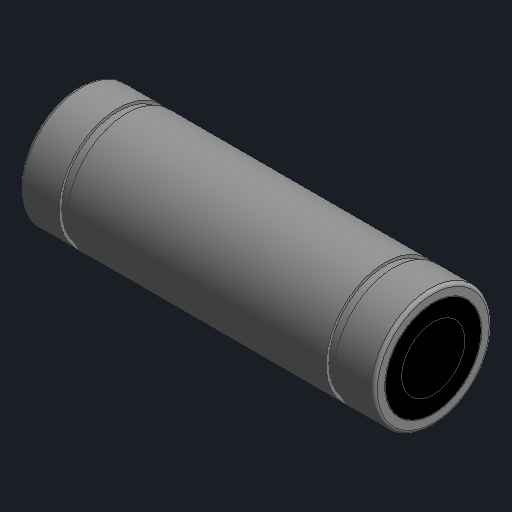
# Autodesk Inventor part: C-LMUW8
Saved by Autodesk Inventor 2022 (Build 260153000, 153)
## iProperties
Category: PARTsolutions
Company: MISUMI
Part Number: C-LMUW8
Material: 一般
Catalog Web Link: www.cadenas.de
Description: ミスミ
Vendor: MISUMI
Document SubType Name: Modeling
Designer: partserver
Manufacturer: MISUMI
Mass: 5.65138 g
Surface Area: 35.5542 cm^2
Volume: 5.65138 cm^3
Density: 1 g/cm^3
Appearance: PSOLRGB-175-175-175
PSOL_IDENT_0: {$CADENAS_DATA\23d-libs\misumi\metric\04_linear_bushings\04_cn\c_lmuw.prj},165 {VTYP=3D},{NB=C-LMUW8
PSOL_IDENT_1: },{LINA=C-LMUW8},{NN=C-LMUW, C-LMUWM},{DATE=01.06.2021 05:20:37},{GEOMDATE=25.09.2019 05:13:57},{VER
PSOL_IDENT_2: SION=},{LINEID=40},{WBVAR=ST},{WBNUMERIC=}  {NB=C-LMUW8},{LINA=C-LMUW8},{KT=DUMMY},{PN=C-LMUW8},{TYP
PSOL_IDENT_3: E=C-LMUW},{ST=},{DDRR=8},{D=15},{L=45},{B=32.8},{BALG=32.8},{W=1.1},{WALG=1.1},{D1=14.3},{D1ALG=14.3
PSOL_IDENT_4: },{R=0.400}
NB: C-LMUW8
NN: C-LMUW, C-LMUWM
NT: C-VALUE Linear Bushings - Double
NBSYN: $PN.
LINA: C-LMUW8
CATALOG: Misumi
PN: C-LMUW8
ST: -
DDRR: 8
D: 15
L: 45
B: 32.8
W: 1.1
D1: 14.3
SUPPLIER: MISUMI
ARTICLENO: C-LMUW8
BOMINFO: C-LMUW8
CREATOR: CADENAS GmbH
Title: C-LMUW8
Author: Cadenas PARTsolutions
Comments: C-VALUE Linear Bushings - Double
Autodesk Inventor part; units mm, degrees
ref_plane "YZ Plane" through (0, 0, 0) normal (1, 0, 0) x (0, 1, 0)
ref_plane "XZ Plane" through (0, 0, 0) normal (0, 1, 0) x (-1, 0, 0)
ref_plane "XY Plane" through (0, 0, 0) normal (0, 0, 1) x (1, 0, 0)
sketch "Sketch_1" plane through (0, 0, 0) normal (0, 0, 1) x (1, 0, 0)
  line L0 (22.5, 0) -> (0, 0)
  line L1 (-22.5, 7.1) -> (-22.5, 6.15)
  line L2 (-22.5, 6.15) -> (-22.45, 6.15)
  line L3 (-22.45, 6.15) -> (-22.45, 6.1)
  line L4 (-22.45, 6.1) -> (22.45, 6.1)
  line L5 (22.45, 6.1) -> (22.45, 6.15)
  line L6 (22.45, 6.15) -> (22.5, 6.15)
  line L7 (22.5, 6.15) -> (22.5, 7.1)
  arc A0 (22.5, 7.1) -> (22.1, 7.5) centre (22.1, 7.1) ccw
  line L8 (22.1, 7.5) -> (17.5, 7.5)
  line L9 (17.5, 7.5) -> (17.5, 7.15)
  line L10 (17.5, 7.15) -> (16.4, 7.15)
  line L11 (16.4, 7.15) -> (16.4, 7.5)
  line L12 (16.4, 7.5) -> (-16.4, 7.5)
  line L13 (-16.4, 7.5) -> (-16.4, 7.15)
  line L14 (-16.4, 7.15) -> (-17.5, 7.15)
  line L15 (-17.5, 7.15) -> (-17.5, 7.5)
  line L16 (-17.5, 7.5) -> (-22.1, 7.5)
  arc A1 (-22.1, 7.5) -> (-22.5, 7.1) centre (-22.1, 7.1) ccw
  constraints: 34 end point, 4 point on circle, 2 centre point
revolve "Revolution1" add sketch "Sketch_1" angle 360 about axis through (22.5, 0, 0) along (1, 0, 0)
sketch "Sketch_3" plane through (0, 0, 0) normal (0, 0, 1) x (1, 0, 0)
  line L0 (22.5, 0) -> (0, 0)
  line L1 (-22.5, 6.1) -> (-22.5, 4)
  line L2 (-22.5, 4) -> (22.5, 4)
  line L3 (22.5, 4) -> (22.5, 6.1)
  line L4 (22.5, 6.1) -> (-22.5, 6.1)
  constraints: 10 end point
revolve "Revolution2" add sketch "Sketch_3" angle 360 about axis through (22.5, 0, 0) along (1, 0, 0)
body "Solid1"
